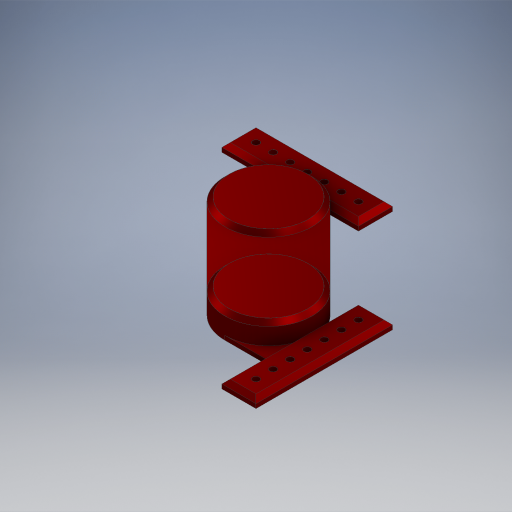
# Autodesk Inventor part: MK3-Swerve-Top-Cover
Saved by Autodesk Inventor 2024.2 (Build 282272000, 272)
## iProperties
Created: 2024-02-25
Part Number: MK3-Swerve-Top-Cover
Material: Generic
Document SubType Name: Modeling
Designer: rohan
Density: 1 g/cm^3
Appearance: Default
Author: rohan
Autodesk Inventor part; units mm, degrees
ref_plane "YZ Plane" through (0, 0, 0) normal (1, 0, 0) x (0, 1, 0)
ref_plane "XZ Plane" through (0, 0, 0) normal (0, 1, 0) x (-1, 0, 0)
ref_plane "XY Plane" through (0, 0, 0) normal (0, 0, 1) x (1, 0, 0)
sketch "Sketch1" plane through (0, 0, 0) normal (0, 1, 0) x (-1, 0, 0)
  circle A0 centre (0, 0) radius 29.21
  circle A1 centre (57.4802, -57.4802) radius 29.21
  circle A2 centre (0, 0) radius 32.385
  circle A3 centre (57.4802, -57.4802) radius 32.385
  dimension "d0" = 58.42
  dimension "d1" = 58.42
  dimension "d2" = 57.4802
  dimension "d3" = 57.4802
  dimension "d4" = 3.175
  dimension "d5" = 3.175
  constraints: 4 centre point, 1 coincident
  measures "d0" diameter of A0
  measures "d1" diameter of A1
  measures "d2" horizontal distance of A1.centre point (0, 0)
  measures "d3" horizontal distance of A1.centre point (0, 0)
  measures "d4" radial gap between concentric circles of A0 A2
  measures "d5" radial gap between concentric circles of A1 A3
extrude "Extrusion1" add sketch "Sketch1" against normal blind 14.8844
sketch "Sketch2" plane through (0, 0, 0) normal (0, 1, 0) x (1, 0, 0)
  circle A0 centre (0, 0) radius 32.385 projected
  circle A1 centre (0, 0) radius 29.21 projected
  circle A2 centre (-57.4802, 57.4802) radius 32.385 projected
  circle A3 centre (-57.4802, 57.4802) radius 29.21 projected
extrude "Extrusion2" add sketch "Sketch2" along normal blind 0.762
sketch "Sketch3" plane through (0, 0.762, 0) normal (0, 1, 0) x (1, 0, 0)
  circle A0 centre (0, 0) radius 32.385 projected
  circle A1 centre (0, 0) radius 29.21 projected
  circle A2 centre (-57.4802, 57.4802) radius 32.385 projected
  circle A3 centre (-57.4802, 57.4802) radius 29.21 projected
extrude "Extrusion3" add sketch "Sketch3" along normal blind 3.175 contours A0 | A1 | A2 | A3
chamfer "Chamfer1" distance 3.175 angle 45 2 edges at (-32.385, 3.937, 0) (-89.8652, 3.937, -57.4802)
sketch "Sketch4" plane through (0, -14.8844, 0) normal (0, -1, 0) x (1, 0, 0)
  line L0 (55.499, 64.42) -> (55.499, -12.6433)
  circle A0 centre (0, 0) radius 29.21 projected
  circle A1 centre (-57.4802, -57.4802) radius 29.21 projected
  line L1 (55.499, -36.7792) -> (55.499, -12.6433)
  line L2 (55.499, -36.7792) -> (30.099, -36.7792)
  line L3 (30.099, -36.7792) -> (30.099, 64.8208)
  line L4 (30.099, 64.8208) -> (55.499, 64.8208)
  line L5 (55.499, 64.8208) -> (55.499, 64.42)
  line L6 (-20.701, -112.9792) -> (-20.701, -87.5792)
  line L7 (-20.701, -87.5792) -> (-122.301, -87.5792)
  line L8 (-122.301, -87.5792) -> (-122.301, -112.9792)
  line L9 (-122.301, -112.9792) -> (-20.701, -112.9792)
  circle A2 centre (42.799, -24.0792) radius 2.4892
  circle A3 centre (42.799, -11.3792) radius 2.4892
  circle A4 centre (42.799, 1.3208) radius 2.4892
  circle A5 centre (42.799, 14.0208) radius 2.4892
  circle A6 centre (42.799, 26.7208) radius 2.4892
  circle A7 centre (42.799, 39.4208) radius 2.4892
  circle A8 centre (42.799, 52.1208) radius 2.4892
  circle A9 centre (-33.401, -100.2792) radius 2.4892
  circle A10 centre (-46.101, -100.2792) radius 2.4892
  circle A11 centre (-58.801, -100.2792) radius 2.4892
  circle A12 centre (-71.501, -100.2792) radius 2.4892
  circle A13 centre (-84.201, -100.2792) radius 2.4892
  circle A14 centre (-96.901, -100.2792) radius 2.4892
  circle A15 centre (-109.601, -100.2792) radius 2.4892
  point P0 (-20.701, -100.2792)
  dimension "d16" = 55.499
  dimension "d18" = 36.7792
  dimension "d19" = 55.499
  dimension "d20" = 25.4
  dimension "d21" = 101.6
  dimension "d26" = 36.7792
  dimension "d27" = 55.499
  dimension "d28" = 25.4
  dimension "d29" = 101.6
  dimension "d30" = 4.9784
  dimension "d31" = 12.7
  dimension "d32" = 12.7
  dimension "d35" = 12.7
  dimension "d40" = 4.9784
  dimension "d41" = 12.7
  dimension "d42" = 12.7
  dimension "d45" = 12.7
  constraints: 20 end point, 14 centre point, 5 perpendicular, 4 vertical, 2 horizontal, 1 midpoint, 24 other
  measures "d16" distance from line of A0.centre L0
  measures "d18" vertical distance of A0.centre L1.start
  measures "d19" horizontal distance of L1.start A0.centre
  measures "d20" distance of L1.start L2.end
  measures "d21" distance of L2.end L3.end
  measures "d26" horizontal distance of L6.start A1.centre
  measures "d27" vertical distance of L6.start A1.centre
  measures "d28" distance of L6.start L6.end
  measures "d29" distance of L6.end L7.end
  measures "d30" diameter of A2
  measures "d31" distance from line of A2.centre L2
  measures "d32" distance from line of A2.centre L1
  measures "d35" distance of A2.centre A3.centre
  measures "d40" diameter of A9
  measures "d41" distance of A9.centre point (-20.701, -100.279)
  measures "d42" distance from line of L9 A9.centre
  measures "d45" distance of A9.centre A10.centre
extrude "Extrusion4" add sketch "Sketch4" against normal blind 6.35 contours L0 L1 L2 L3 L4 L5 | L9 L8 L7 L6
chamfer "Chamfer2" distance 3.175 angle 45 8 edges at (30.099, -8.5344, 38.3862) (42.799, -8.5344, 64.8208) (55.499, -8.5344, 14.0208) (42.799, -8.5344, -36.7792) (-20.701, -8.5344, -100.2792) (-33.1148, -8.5344, -87.5792) (-71.501, -8.5344, -112.9792) (-122.301, -8.5344, -100.2792)
sketch "Sketch5" plane through (0, -14.8844, 0) normal (0, -1, 0) x (1, 0, 0)
  circle A0 centre (42.799, -24.0792) radius 2.4892 projected
  circle A1 centre (42.799, -11.3792) radius 2.4892 projected
  circle A2 centre (42.799, 1.3208) radius 2.4892 projected
  circle A3 centre (42.799, 14.0208) radius 2.4892 projected
  circle A4 centre (42.799, 26.7208) radius 2.4892 projected
  circle A5 centre (42.799, 39.4208) radius 2.4892 projected
  circle A6 centre (42.799, 52.1208) radius 2.4892 projected
  circle A7 centre (0, 0) radius 29.21 projected
  arc A8 (30.099, 11.9515) -> (30.099, -11.9515) centre (0, 0) ccw projected
  line L0 (30.099, -11.9515) -> (30.099, -36.7792) projected
  line L1 (30.099, -36.7792) -> (55.499, -36.7792) projected
  line L2 (55.499, -36.7792) -> (55.499, 64.8208) projected
  line L3 (55.499, 64.8208) -> (30.099, 64.8208) projected
  line L4 (30.099, 64.8208) -> (30.099, 11.9515) projected
  circle A9 centre (-109.601, -100.2792) radius 2.4892 projected
  circle A10 centre (-84.201, -100.2792) radius 2.4892 projected
  circle A11 centre (-58.801, -100.2792) radius 2.4892 projected
  circle A12 centre (-33.401, -100.2792) radius 2.4892 projected
  circle A13 centre (-46.101, -100.2792) radius 2.4892 projected
  circle A14 centre (-71.501, -100.2792) radius 2.4892 projected
  circle A15 centre (-96.901, -100.2792) radius 2.4892 projected
  arc A16 (-45.5287, -87.5792) -> (-69.4317, -87.5792) centre (-57.4802, -57.4802) ccw projected
  line L5 (-69.4317, -87.5792) -> (-122.301, -87.5792) projected
  line L6 (-122.301, -87.5792) -> (-122.301, -112.9792) projected
  line L7 (-122.301, -112.9792) -> (-20.701, -112.9792) projected
  line L8 (-20.701, -112.9792) -> (-20.701, -87.5792) projected
  line L9 (-20.701, -87.5792) -> (-45.5287, -87.5792) projected
  circle A17 centre (-57.4802, -57.4802) radius 29.21 projected
  circle A18 centre (-57.4802, -57.4802) radius 32.385 projected
  circle A19 centre (0, 0) radius 32.385 projected
  line L10 (-34.5805, -80.3799) -> (22.8997, -22.8997)
  line L11 (-22.8997, 22.8997) -> (-80.3799, -34.5805)
  arc A20 (30.099, 11.9515) -> (30.099, -11.9515) centre (0, 0) ccw projected
  point P0 (22.8997, -22.8997)
  constraints: 4 end point, 4 point on circle, 4 tangent
extrude "Extrusion5" add sketch "Sketch5" against normal blind 15.6464 contours A8 L10 A16 L11
sketch "Sketch6" plane through (0, -14.8844, 0) normal (0, -1, 0) x (1, 0, 0)
  circle A0 centre (-57.4802, -57.4802) radius 29.21 projected
  circle A1 centre (-96.901, -100.2792) radius 2.4892 projected
  circle A2 centre (-71.501, -100.2792) radius 2.4892 projected
  circle A3 centre (-46.101, -100.2792) radius 2.4892 projected
  circle A4 centre (-33.401, -100.2792) radius 2.4892 projected
  circle A5 centre (-58.801, -100.2792) radius 2.4892 projected
  circle A6 centre (-84.201, -100.2792) radius 2.4892 projected
  circle A7 centre (-109.601, -100.2792) radius 2.4892 projected
  circle A8 centre (42.799, -24.0792) radius 2.4892 projected
  circle A9 centre (42.799, -11.3792) radius 2.4892 projected
  circle A10 centre (42.799, 1.3208) radius 2.4892 projected
  circle A11 centre (42.799, 14.0208) radius 2.4892 projected
  circle A12 centre (42.799, 26.7208) radius 2.4892 projected
  circle A13 centre (42.799, 39.4208) radius 2.4892 projected
  circle A14 centre (42.799, 52.1208) radius 2.4892 projected
  circle A15 centre (0, 0) radius 29.21 projected
  arc A16 (30.099, 11.9515) -> (-22.8997, 22.8997) centre (0, 0) ccw projected
  line L0 (-22.8997, 22.8997) -> (-80.3799, -34.5805) projected
  arc A17 (-80.3799, -34.5805) -> (-69.4317, -87.5792) centre (-57.4802, -57.4802) ccw projected
  line L1 (-69.4317, -87.5792) -> (-122.301, -87.5792) projected
  line L2 (-122.301, -87.5792) -> (-122.301, -112.9792) projected
  line L3 (-122.301, -112.9792) -> (-20.701, -112.9792) projected
  line L4 (-20.701, -112.9792) -> (-20.701, -87.5792) projected
  line L5 (-20.701, -87.5792) -> (-45.5287, -87.5792) projected
  arc A18 (-45.5287, -87.5792) -> (-34.5805, -80.3799) centre (-57.4802, -57.4802) ccw projected
  line L6 (-34.5805, -80.3799) -> (22.8997, -22.8997) projected
  arc A19 (22.8997, -22.8997) -> (30.099, -11.9515) centre (0, 0) ccw projected
  line L7 (30.099, -11.9515) -> (30.099, -36.7792) projected
  line L8 (30.099, -36.7792) -> (55.499, -36.7792) projected
  line L9 (55.499, -36.7792) -> (55.499, 64.8208) projected
  line L10 (55.499, 64.8208) -> (30.099, 64.8208) projected
  line L11 (30.099, 64.8208) -> (30.099, 11.9515) projected
  arc A20 (22.8997, -22.8997) -> (-22.8997, 22.8997) centre (0, 0) ccw projected
  line L12 (0, 32.385) -> (30.099, 32.385)
  line L13 (-89.8652, -57.4802) -> (-89.8652, -87.5792)
  arc A21 (-80.3799, -34.5805) -> (-34.5805, -80.3799) centre (-57.4802, -57.4802) ccw projected
  constraints: 4 end point, 4 tangent, 2 perpendicular, 2 point on circle, 2 point on line
extrude "Extrusion6" add sketch "Sketch6" against normal blind 3.175 contours A16 L12 L11 | A17 L1 L13
body "Solid1"
